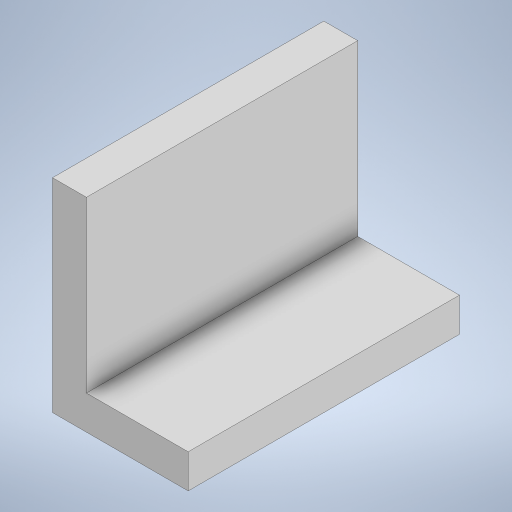
# Autodesk Inventor part: LPart
Saved by Autodesk Inventor 2023 (Build 270158000, 158)
## iProperties
Created: 2025-04-08
Part Number: LPart
Material: Generic
Document SubType Name: Modeling
Designer: gsunkari
Density: 1 g/cm^3
Appearance: Default
Author: gsunkari
Autodesk Inventor part; units mm, degrees
ref_plane "YZ Plane" through (0, 0, 0) normal (1, 0, 0) x (0, 1, 0)
ref_plane "XZ Plane" through (0, 0, 0) normal (0, 1, 0) x (-1, 0, 0)
ref_plane "XY Plane" through (0, 0, 0) normal (0, 0, 1) x (1, 0, 0)
sketch "Sketch1" plane through (0, 0, 0) normal (0, 0, 1) x (1, 0, 0)
  line L0 (0, 0) -> (2540, 0)
  line L1 (2540, 0) -> (2540, 635)
  line L2 (2540, 635) -> (635, 635)
  line L3 (635, 635) -> (635, 3810)
  line L4 (635, 3810) -> (0, 3810)
  line L5 (0, 3810) -> (0, 0)
  dimension "d3" = 3810
  dimension "d4" = 2540
  dimension "d5" = 635
  dimension "d6" = 1905
  constraints: 12 end point, 5 perpendicular, 1 horizontal
  measures "d3" distance of L4.end L0.start
  measures "d4" distance of L0.start L0.end
  measures "d5" distance of L0.end L1.end
  measures "d6" distance of L1.end L2.end
extrude "Extrusion1" add sketch "Sketch1" along normal blind 5080
equation "\"Thickness\" = d5"
body "Solid1"
